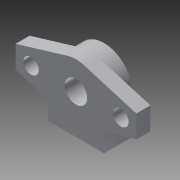
# Autodesk Inventor part: shf8
Saved by Autodesk Inventor 2014 (Build 180170000, 170)
## iProperties
Created: 2014-07-14
Part Number: shf8
Material: Generic
Document SubType Name: Modeling
Designer: cruiser
Density: 1 g/cm^3
Appearance: Aluminum - Flat
Author: cruiser
Autodesk Inventor part; units mm, degrees
ref_plane "YZ Plane" through (0, 0, 0) normal (1, 0, 0) x (0, 1, 0)
ref_plane "XZ Plane" through (0, 0, 0) normal (0, 1, 0) x (-1, 0, 0)
ref_plane "XY Plane" through (0, 0, 0) normal (0, 0, 1) x (1, 0, 0)
sketch "Sketch1" plane through (0, 0, 0) normal (0, 1, 0) x (-1, 0, 0)
  circle A0 centre (0, 0) radius 4
  circle A1 centre (0, 0) radius 10
  circle A2 centre (-16, 0) radius 2.75
  line L0 (21.5, -4) -> (-21.5, -4)
  line L1 (-21.5, -4) -> (-21.5, 4)
  line L2 (-21.5, 4) -> (21.5, 4)
  line L3 (21.5, 4) -> (21.5, -4)
  line L4 (21.5, -4) -> (-21.5, 4) construction
  line L5 (-21.5, -4) -> (21.5, 4) construction
  line L6 (21.5, 0) -> (-21.5, 0)
  circle A3 centre (16, 0) radius 2.75
  line L7 (0, 10) -> (0, -14)
  line L8 (-21.5, 4) -> (-2.8689, 9.5796)
  line L9 (21.5, 4) -> (2.8689, 9.5796)
  line L10 (21.5, -4) -> (2.8689, -9.5796)
  line L11 (-21.5, -4) -> (-2.8689, -9.5796)
  line L12 (-10, -14) -> (10, -14)
  line L13 (10, -14) -> (10, -4)
  line L14 (10, 0) -> (-10, 0)
  line L15 (-10, -4) -> (-10, -14)
  dimension "d0" = 8
  dimension "d1" = 20
  dimension "d2" = 5.5
  dimension "d3" = 43
  dimension "d4" = 8
  dimension "d5" = 16
  dimension "d6" = 5.5
  dimension "d7" = 16
  dimension "d8" = 24
  dimension "d9" = 0
  dimension "d10" = 10
  constraints: 32 end point, 5 midpoint, 5 parallel, 5 point on circle, 5 point on line, 4 centre point, 3 perpendicular, 3 tangent, 2 coincident, 2 horizontal
  measures "d0" diameter of A0
  measures "d1" diameter of A1
  measures "d2" diameter of A2
  measures "d3" distance of L1.end L2.end
  measures "d4" distance of L0.end L1.end
  measures "d5" distance of point (0, 0) A2.centre
  measures "d6" diameter of A3
  measures "d7" distance of point (0, 0) A3.centre
  measures "d8" distance of L7.end L7.start
  measures "d9" distance from line of point (0, 0) L7
  measures "d10" distance from line of L13 A1.centre
extrude "Extrusion1" add sketch "Sketch1" along normal blind 5 contours L6 A1 L0 A0 | A0 L2 A1 L6 | A0 L6 A1 L2 | L7 A1 L2 | L2 A1 L7 | L0 A1 L6 A0 | L7 A1 L0 | L0 A1 L7 | L6 A3 L3 L0 A1 | A1 L2 L3 L6 A3 | L2 L8 A1 | A1 L6 A2 L1 L2 | A1 L9 L2 | L0 L13 L10 A1 | L0 L1 L6 A2 A1 | A1 L11 L15 L0 | L7 L12 L15 L11 A1 | A1 L10 L13 L12 L7 | L0 L10 L13 | L15 L11 L0
sketch "Sketch2" plane through (0, 5, 0) normal (0, 1, 0) x (1, 0, 0)
  circle A0 centre (0, 0) radius 4 projected
  arc A1 (-10, 0) -> (10, 0) centre (0, 0) ccw
  line L0 (-10, 14) -> (10, 14)
  line L1 (10, 14) -> (10, 0)
  line L2 (-10, 0) -> (-10, 14)
  circle A2 centre (0, 0) radius 4
  dimension "d13" = 20
  dimension "d15" = 20
  constraints: 6 end point, 2 centre point, 2 coincident, 2 point on circle, 1 concentric, 1 horizontal, 1 parallel, 1 perpendicular
  measures "d13" diameter of A1
  measures "d15" distance between parallel lines of L2 L1
extrude "Extrusion2" add sketch "Sketch2" along normal blind 5
body "Solid1"
